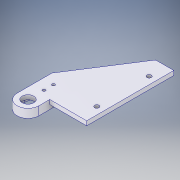
# Autodesk Inventor part: exShort
Saved by Autodesk Inventor 2017 (Build 210142000, 142)
## iProperties
Created: 2017-03-10
Part Number: exShort
Material: Generic
Document SubType Name: Modeling
Designer: Naga
Density: 1 g/cm^3
Appearance: Cool White
Author: Naga
Autodesk Inventor part; units mm, degrees
ref_plane "YZ Plane" through (0, 0, 0) normal (1, 0, 0) x (0, 1, 0)
ref_plane "XZ Plane" through (0, 0, 0) normal (0, 1, 0) x (-1, 0, 0)
ref_plane "XY Plane" through (0, 0, 0) normal (0, 0, 1) x (1, 0, 0)
sketch "Sketch3" plane through (0, 0, 0) normal (0, 1, 0) x (-1, 0, 0)
  line L0 (0, 0) -> (0, -60)
  line L1 (0, 0) -> (60, 0) construction
  line L2 (0, -60) -> (12.519, -60)
  line L3 (0, 0) -> (25.4, 0)
  line L4 (25.4, 0) -> (25.4, 7.5)
  arc A0 (40.4, 7.5) -> (25.4, 7.5) centre (32.9, 7.5) ccw
  line L5 (40.4, 7.5) -> (40.4, -16.519)
  line L6 (40.4, -16.519) -> (12.519, -60)
  line L7 (0, -30) -> (5, -30)
  line L8 (5, -60) -> (5, -48)
  line L9 (5, 0) -> (5, -12)
  circle A1 centre (5, -12) radius 1.5
  circle A2 centre (5, -48) radius 1.5
  circle A3 centre (32.9, 7.5) radius 4
  line L10 (32.9, 7.5) -> (32.9, -3.512)
  line L11 (32.9, -3.512) -> (32.9, -10.02)
  circle A4 centre (32.9, -3.512) radius 1
  circle A5 centre (32.9, -10.02) radius 1
  dimension "d6" = 60
  dimension "d7" = 90
  dimension "d8" = 12.519
  dimension "d9" = 25.4
  dimension "d10" = 7.5
  dimension "d11" = 15
  dimension "d13" = 24.019
  dimension "d18" = 5
  dimension "d19" = 12
  dimension "d20" = 12
  dimension "d21" = 3
  dimension "d22" = 3
  dimension "d25" = 8
  dimension "d26" = 11.012
  dimension "d27" = 6.508
  dimension "d28" = 2
  dimension "d29" = 2
  constraints: 24 end point, 6 centre point, 6 vertical, 5 coincident, 3 horizontal, 3 point on line, 2 perpendicular, 2 point on circle, 1 midpoint, 1 tangent
  measures "d6" distance of L0.start L0.end
  measures "d7" angle of L0 L1
  measures "d8" distance of L0.end L2.end
  measures "d9" distance of L0.start L3.end
  measures "d10" distance of L3.end L4.end
  measures "d11" distance of L5.start L4.end
  measures "d13" distance of L5.start L5.end
  measures "d18" distance of L7.start L7.end
  measures "d19" distance of L8.start L8.end
  measures "d20" distance of L9.start L9.end
  measures "d21" diameter of A1
  measures "d22" diameter of A2
  measures "d25" diameter of A3
  measures "d26" distance of L10.start L10.end
  measures "d27" distance of L10.end L11.end
  measures "d28" diameter of A4
  measures "d29" diameter of A5
extrude "Extrusion1" add sketch "Sketch3" along normal blind 3
sketch "Sketch6" plane through (0, 3, 0) normal (0, 1, 0) x (1, 0, 0)
  circle A0 centre (-32.9, -7.5) radius 4 projected
  circle A1 centre (-5, 48) radius 1.5 projected
  circle A2 centre (-5, 12) radius 1.5 projected
  circle A3 centre (-32.9, 10.02) radius 1 projected
  circle A4 centre (-32.9, 3.512) radius 1 projected
  line L0 (0, 0) -> (0, 60) projected
  line L1 (0, 60) -> (-12.519, 60) projected
  line L2 (-12.519, 60) -> (-40.4, 16.519) projected
  line L3 (-40.4, 16.519) -> (-40.4, -7.5) projected
  arc A5 (-40.4, -7.5) -> (-25.4, -7.5) centre (-32.9, -7.5) ccw projected
  line L4 (-25.4, -7.5) -> (-25.4, 0) projected
  line L5 (-25.4, 0) -> (0, 0) projected
  line L6 (-40.4, 16.519) -> (-25.4, 16.519)
  line L7 (-25.4, -7.5) -> (-25.4, 0) projected
  line L8 (-25.4, 16.519) -> (-25.4, 0)
  circle A6 centre (-32.9, -7.5) radius 5.5
  line L9 (-32.9, 10.02) -> (-32.9, 11.52)
  circle A7 centre (-32.9, 11.52) radius 3
  line L10 (-38.4, -7.5) -> (-38.4, -4.5)
  line L11 (-27.4, -7.5) -> (-27.4, -4.5)
  line L12 (-27.4, -4.5) -> (-29.9349, 11.9762)
  line L13 (-38.4, -4.5) -> (-35.8651, 11.9762)
  point P0 (0, 0)
  dimension "d31" = 11
  dimension "d32" = 1.5
  dimension "d33" = 6
  dimension "d34" = 3
  constraints: 14 end point, 4 point on circle, 4 tangent, 3 vertical, 2 centre point, 2 coincident, 1 horizontal, 1 perpendicular
  measures "d31" diameter of A6
  measures "d32" distance of L9.start L9.end
  measures "d33" diameter of A7
  measures "d34" distance of L10.start L10.end
extrude "Extrusion3" add sketch "Sketch6" against normal blind 6 contours L4 A5 L3 L6 L8
body "Solid1"
